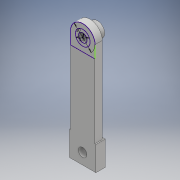
# Autodesk Inventor part: connecting-rod-40
Saved by Autodesk Inventor 2018 (Build 220112000, 112)
## iProperties
Created: 2025-09-15
Part Number: connecting-rod-40
Material: Generic
Document SubType Name: Modeling
Designer: neo
Density: 1 g/cm^3
Appearance: Default
Author: neo
Autodesk Inventor part; units mm, degrees
ref_plane "YZ Plane" through (0, 0, 0) normal (1, 0, 0) x (0, 1, 0)
ref_plane "XZ Plane" through (0, 0, 0) normal (0, 1, 0) x (-1, 0, 0)
ref_plane "XY Plane" through (0, 0, 0) normal (0, 0, 1) x (1, 0, 0)
sketch "Sketch1" plane through (0, 0, 0) normal (0, 1, 0) x (-1, 0, 0)
  circle A0 centre (0, 0) radius 1.75
  arc A1 (5, 0) -> (-5, 0) centre (0, 0) ccw
  circle A2 centre (0, 0) radius 3
  line L0 (5, 0) -> (5, -5)
  line L1 (5, -5) -> (-5, -5)
  line L2 (-5, 0) -> (-5, -5)
  dimension "d0" = 3.5
  dimension "d1" = 10
  dimension "d2" = 6
  constraints: 6 end point, 3 centre point, 3 coincident, 2 perpendicular, 2 point on circle, 2 tangent, 1 vertical
  measures "d0" diameter of A0
  measures "d1" diameter of A1
  measures "d2" diameter of A2
extrude "Extrusion1" add sketch "Sketch1" along normal blind 3 contours L0 L1 L2 A1
extrude "bearing-distance-holder" add sketch "Sketch1" along normal blind 6 contours A2
sketch "Sketch2" plane through (5, 0, -5) normal (0, 0, -1) x (-1, 0, 0)
  line L0 (0, 0) -> (10, 0) projected
  line L1 (10, 0) -> (10, 3) projected
  line L2 (0, 3) -> (10, 3) projected
  line L3 (0, 0) -> (0, 3) projected
  point P0 (5, 0)
extrude "L" add sketch "Sketch2" along normal blind 40
sketch "Sketch6" plane through (5, 0, -45) normal (0, 0, -1) x (-1, 0, 0)
  line L0 (10.4, 3.8) -> (-0.4, 3.8)
  line L1 (-0.4, 3.8) -> (-0.4, 0)
  line L2 (-0.4, 0) -> (10.4, 0)
  line L3 (10.4, 0) -> (10.4, 3.8)
  line L4 (10, 0) -> (10, 3) projected
  line L5 (0, 0) -> (10, 0) projected
  line L6 (10, 3) -> (0, 3) projected
  line L7 (0, 3) -> (0, 0) projected
  point P0 (5, 0)
  dimension "d20" = 0.4
  dimension "d21" = 0
  dimension "d22" = 0.8
  dimension "d23" = 0.4
  constraints: 8 end point, 2 parallel, 1 horizontal, 1 perpendicular
  measures "d20" distance between parallel lines of L4 L3
  measures "d21" distance between parallel lines of L5 L2
  measures "d22" distance between parallel lines of L6 L0
  measures "d23" distance between parallel lines of L7 L1
extrude "Extrusion7" add sketch "Sketch6" against normal blind 10 contours L3 L2 L4 L6 L7 L1 L0
sketch "Sketch5" plane through (0, 3.8, 0) normal (0, 1, 0) x (1, 0, 0)
  circle A0 centre (0, 40.5) radius 1.75
  line L0 (-5, 45) -> (5, 45) projected
  point P0 (0, 0)
  dimension "d16" = 4.5
  dimension "d17" = 3.5
  constraints: 1 centre point
  measures "d16" distance from line of L0 A0.centre
  measures "d17" diameter of A0
extrude "Extrusion8" cut sketch "Sketch5" along normal mid plane 10
body "Solid1"
